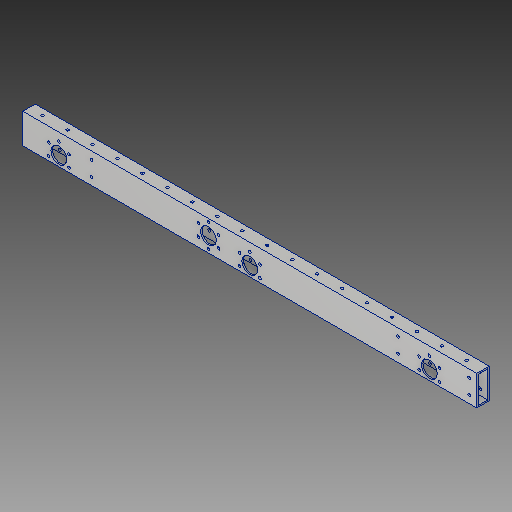
# Autodesk Inventor part: Main Extrusion
Saved by Autodesk Inventor 2019.4 (Build 234330000, 330)
## iProperties
Created: 2020-01-05
Part Number: Main Extrusion
Material: Aluminum 6061
Document SubType Name: Modeling
Designer: Mark
Mass: 1095.18 g
Surface Area: 2784.42 cm^2
Volume: 405.623 cm^3
Density: 2.7 g/cm^3
Appearance: Aluminum - Flat
Author: Mark
Autodesk Inventor part; units mm, degrees
ref_plane "YZ Plane" through (0, 0, 0) normal (1, 0, 0) x (0, 1, 0)
ref_plane "XZ Plane" through (0, 0, 0) normal (0, 1, 0) x (-1, 0, 0)
ref_plane "XY Plane" through (0, 0, 0) normal (0, 0, 1) x (1, 0, 0)
sketch "Sketch1" plane through (0, 0, 0) normal (1, 0, 0) x (0, 1, 0)
  line L0 (-30, 12.5) -> (30, 12.5)
  line L1 (30, 12.5) -> (30, -12.5)
  line L2 (30, -12.5) -> (-30, -12.5)
  line L3 (-30, -12.5) -> (-30, 12.5)
  line L4 (-30, 12.5) -> (30, -12.5) construction
  line L5 (30, 12.5) -> (-30, -12.5) construction
  line L6 (-27, 9.5) -> (27, 9.5)
  line L7 (27, 9.5) -> (27, -9.5)
  line L8 (27, -9.5) -> (-27, -9.5)
  line L9 (-27, -9.5) -> (-27, 9.5)
  line L10 (-27, 9.5) -> (27, -9.5) construction
  line L11 (27, 9.5) -> (-27, -9.5) construction
  point P0 (0, 0)
  dimension "d0" = 60
  dimension "d1" = 25
  dimension "d2" = 54
  dimension "d3" = 19
  constraints: 24 end point, 4 midpoint, 4 parallel, 2 horizontal, 2 perpendicular
  measures "d0" distance of L1.end L2.end
  measures "d1" distance of L0.end L1.end
  measures "d2" distance of L7.end L8.end
  measures "d3" distance of L6.end L7.end
extrude "Extrusion1" add sketch "Sketch1" along normal blind 910
sketch "Sketch2" plane through (0, -30, 12.5) normal (0, 0, 1) x (1, 0, 0)
  circle A0 centre (455, 20) radius 16
  circle A1 centre (72.3744, 20) radius 16
  circle A2 centre (815, 20) radius 16
  line L0 (0, 0) -> (0, 60) projected
  line L1 (0, 0) -> (910, 0) projected
  circle A3 centre (372.2077, 30) radius 16
  circle A4 centre (455, 20) radius 23.5 construction
  line L2 (455, 20) -> (455, -3.5) construction
  line L3 (455, 20) -> (478.5, 20) construction
  circle A5 centre (455, -3.5) radius 2.75
  circle A6 centre (475.3516, 8.25) radius 2.75
  circle A7 centre (475.3516, 31.75) radius 2.75
  circle A8 centre (455, 43.5) radius 2.75
  circle A9 centre (434.6484, 31.75) radius 2.75
  circle A10 centre (434.6484, 8.25) radius 2.75
  circle A11 centre (372.2077, 30) radius 23.5 construction
  line L4 (372.2077, 30) -> (372.2077, 6.5) construction
  line L5 (372.2077, 30) -> (395.7077, 30) construction
  circle A12 centre (392.5593, 18.25) radius 2.75
  circle A13 centre (392.5593, 41.75) radius 2.75
  circle A14 centre (372.2077, 53.5) radius 2.75
  circle A15 centre (351.8561, 41.75) radius 2.75
  circle A16 centre (351.8561, 18.25) radius 2.75
  circle A17 centre (372.2077, 6.5) radius 2.75
  circle A18 centre (72.3744, 20) radius 23.5 construction
  line L6 (72.3744, 20) -> (72.3744, -3.5) construction
  line L7 (72.3744, 20) -> (95.8744, 20) construction
  circle A19 centre (72.3744, -3.5) radius 2.75
  circle A20 centre (92.726, 8.25) radius 2.75
  circle A21 centre (92.726, 31.75) radius 2.75
  circle A22 centre (72.3744, 43.5) radius 2.75
  circle A23 centre (52.0229, 31.75) radius 2.75
  circle A24 centre (52.0229, 8.25) radius 2.75
  circle A25 centre (815, 20) radius 23.5 construction
  line L8 (815, 20) -> (815, -3.5) construction
  circle A26 centre (815, -3.5) radius 2.75
  circle A27 centre (835.3516, 8.25) radius 2.75
  circle A28 centre (835.3516, 31.75) radius 2.75
  circle A29 centre (815, 43.5) radius 2.75
  circle A30 centre (794.6484, 31.75) radius 2.75
  circle A31 centre (794.6484, 8.25) radius 2.75
  point P0 (0, 30)
  dimension "d22" = 47
  dimension "d36" = 47
  dimension "d43" = 47
  dimension "d6" = 32
  dimension "d7" = 32
  dimension "d8" = 32
  dimension "d9" = 455
  dimension "d10" = 20
  dimension "d13" = 20
  dimension "d14" = 20
  dimension "d18" = 32
  dimension "d19" = 30
  dimension "d20" = 83.394
  dimension "d21" = 300
  dimension "d23" = 90
  dimension "d24" = 5.5
  dimension "d27" = 360
  dimension "d29" = 47
  dimension "d30" = 90
  dimension "d31" = 5.5
  dimension "d34" = 360
  dimension "d37" = 90
  dimension "d38" = 5.5
  dimension "d41" = 360
  dimension "d44" = 360
  dimension "d45" = 5.5
  dimension "d48" = 360
  constraints: 29 centre point, 14 end point, 8 coincident, 3 horizontal, 3 perpendicular, 3 vertical alignment, 2 point on circle, 1 vertical, 58 other
  measures "d6" diameter of A0
  measures "d7" diameter of A1
  measures "d8" diameter of A2
  measures "d9" distance from line of L0 A0.centre
  measures "d10" distance from line of L1 A0.centre
  measures "d13" distance from line of L1 A1.centre
  measures "d14" distance from line of L1 A2.centre
  measures "d18" diameter of A3
  measures "d19" distance from line of L1 A3.centre
  measures "d20" distance of A0.centre A3.centre
  measures "d21" distance of A3.centre A1.centre
  measures "d23" angle of L2 L3
  measures "d24" diameter of A5
  measures "d29" diameter of A11
  measures "d30" angle of L4 L5
  measures "d31" diameter of A12
  measures "d37" angle of L6 L7
  measures "d38" diameter of A19
  measures "d44" distance of A0.centre A2.centre
  measures "d45" diameter of A26
extrude "Extrusion2" cut sketch "Sketch2" against normal blind 30 contours A0 | A1 | A2 | A3 | A6 | A7 | A8 | A9 | A10 | A12 | A13 | A14 | A15 | A16 | A17 | A20 | A21 | A22 | A23 | A24 | A27 | A28 | A29 | A30 | A31
sketch "Sketch3" plane through (0, -30, -12.5) normal (0, -1, 0) x (1, 0, 0)
  circle A0 centre (27.5, 12.5) radius 2.75
  line L0 (0, 25) -> (910, 25) projected
  line L1 (0, 0) -> (0, 25) projected
  circle A1 centre (77.5, 12.5) radius 2.75
  circle A2 centre (127.5, 12.5) radius 2.75
  circle A3 centre (177.5, 12.5) radius 2.75
  circle A4 centre (227.5, 12.5) radius 2.75
  circle A5 centre (277.5, 12.5) radius 2.75
  circle A6 centre (327.5, 12.5) radius 2.75
  circle A7 centre (377.5, 12.5) radius 2.75
  circle A8 centre (427.5, 12.5) radius 2.75
  circle A9 centre (477.5, 12.5) radius 2.75
  circle A10 centre (527.5, 12.5) radius 2.75
  circle A11 centre (577.5, 12.5) radius 2.75
  circle A12 centre (627.5, 12.5) radius 2.75
  circle A13 centre (677.5, 12.5) radius 2.75
  circle A14 centre (727.5, 12.5) radius 2.75
  circle A15 centre (777.5, 12.5) radius 2.75
  circle A16 centre (827.5, 12.5) radius 2.75
  circle A17 centre (877.5, 12.5) radius 2.75
  circle A18 centre (927.5, 12.5) radius 2.75
  circle A19 centre (977.5, 12.5) radius 2.75
  point P0 (0, 12.5)
  dimension "d50" = 5.5
  dimension "d51" = 12.5
  dimension "d52" = 27.5
  dimension "d55" = 50
  constraints: 20 centre point, 1 horizontal, 38 other
  measures "d50" diameter of A0
  measures "d51" distance from line of L0 A0.centre
  measures "d52" distance from line of L1 A0.centre
  measures "d55" distance of A0.centre A1.centre
extrude "Extrusion3" cut sketch "Sketch3" against normal blind 60 contours A0 | A1 | A2 | A3 | A4 | A5 | A6 | A7 | A8 | A9 | A10 | A11 | A12 | A13 | A14 | A15 | A16 | A17
sketch "Sketch4" plane through (0, -30, 12.5) normal (0, 0, 1) x (1, 0, 0)
  circle A0 centre (138, 45) radius 2.75
  line L0 (0, 60) -> (910, 60) projected
  line L1 (0, 0) -> (0, 60) projected
  circle A1 centre (138, 15) radius 2.75
  line L2 (0, 0) -> (910, 0) projected
  circle A2 centre (752, 45) radius 2.75
  circle A3 centre (752, 15) radius 2.75
  circle A4 centre (895, 45) radius 2.75
  circle A5 centre (895, 15) radius 2.75
  line L3 (910, 60) -> (910, 0) projected
  point P0 (0, 30)
  dimension "d62" = 5.5
  dimension "d63" = 15
  dimension "d64" = 138
  dimension "d65" = 5.5
  dimension "d66" = 15
  dimension "d67" = 138
  dimension "d68" = 5.5
  dimension "d69" = 5.5
  dimension "d70" = 5.5
  dimension "d71" = 5.5
  dimension "d72" = 15
  dimension "d73" = 15
  dimension "d74" = 15
  dimension "d75" = 15
  dimension "d76" = 15
  dimension "d77" = 15
  dimension "d78" = 143
  dimension "d79" = 143
  constraints: 6 centre point
  measures "d62" diameter of A0
  measures "d63" distance from line of L0 A0.centre
  measures "d64" distance from line of L1 A0.centre
  measures "d65" diameter of A1
  measures "d66" distance from line of L2 A1.centre
  measures "d67" distance from line of L1 A1.centre
  measures "d68" diameter of A2
  measures "d69" diameter of A3
  measures "d70" diameter of A4
  measures "d71" diameter of A5
  measures "d72" distance from line of L0 A4.centre
  measures "d73" distance from line of L0 A2.centre
  measures "d74" distance from line of L2 A3.centre
  measures "d75" distance from line of L2 A5.centre
  measures "d76" distance from line of L3 A4.centre
  measures "d77" distance from line of L3 A5.centre
  measures "d78" distance of A4.centre A2.centre
  measures "d79" distance of A5.centre A3.centre
extrude "Extrusion4" cut sketch "Sketch4" against normal blind 60 contours A0 | A1 | A2 | A3 | A4 | A5
equation "\"d13\" = d10"
equation "\"d14\" = d10"
equation "\"d66\" = d63"
equation "\"d67\" = d64"
equation "\"d72\" = d63"
equation "\"d73\" = d63"
equation "\"d74\" = d63"
equation "\"d75\" = d63"
equation "\"d77\" = d76"
equation "\"d79\" = d78"
body "Solid1"
